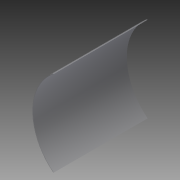
# Autodesk Inventor part: SideRound
Saved by Autodesk Inventor 2014 SP1 (Build 180222100, 222)
## iProperties
Created: 2015-04-12
Part Number: SideRound
Material: PMMA Plastic
Document SubType Name: Modeling
Designer: david
Mass: 220.17 g
Surface Area: 1882.18 cm^2
Volume: 185.328 cm^3
Density: 1.188 g/cm^3
Appearance: Polycarbonate - Clear
Author: david
Autodesk Inventor part; units mm, degrees
ref_plane "YZ Plane" through (0, 0, 0) normal (1, 0, 0) x (0, 1, 0)
ref_plane "XZ Plane" through (0, 0, 0) normal (0, 1, 0) x (-1, 0, 0)
ref_plane "XY Plane" through (0, 0, 0) normal (0, 0, 1) x (1, 0, 0)
sketch "Sketch1" plane through (0, 0, 0) normal (0, 1, 0) x (-1, 0, 0)
  arc A0 (119.8499, -150) -> (119.8499, 150) centre (0, 0) ccw
  line L0 (-197.4383, 150) -> (116.619, 150) construction
  line L1 (-197.4383, -150) -> (116.619, -150) construction
  line L2 (116.619, -150) -> (119.8499, -150)
  line L3 (116.619, 150) -> (119.8499, 150)
  arc A1 (116.619, -150) -> (116.619, 150) centre (0, 0) ccw
  line L4 (0, 0) -> (113.5232, 0) construction
  dimension "d2" = 300
  dimension "d3" = 190
  dimension "d4" = 2
  constraints: 10 end point, 5 point on circle, 4 parallel, 2 centre point, 2 coincident, 2 collinear, 1 horizontal, 1 other
  measures "d2" distance between parallel lines of L1 L0
  measures "d3" radius of A1
  measures "d4" radial gap between concentric circles of A0 A1
extrude "Extrusion1" add sketch "Sketch1" along normal blind 330
equation "\"d2\" = Chassis_Body_Length"
equation "\"d3\" = 0.5 * Chassis_Body_Diameter"
equation "\"d4\" = SideRound_Thickness"
equation "\"Chassis_Body_Length\" = 300"
equation "\"Chassis_Body_Diameter\" = 380"
equation "\"SideRound_Thickness\" = 2"
body "Solid1"
